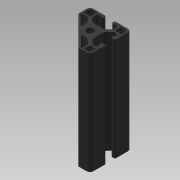
# Autodesk Inventor part: 40-4045-LITE-BLACK-FB
Saved by Autodesk Inventor 2013 (Build 170138000, 138)
## iProperties
Company: 80/20 Inc.
Created: 2014-04-23
Part Number: 40-4045-LITE-BLACK-FB
Material: Generic
Document SubType Name: Modeling
Designer: Ross Bowman
Density: 1 g/cm^3
Engineer: Ross Bowman
Catalog Web Link: 8020.net
Vendor: 80/20 Inc.
Material: 6105-T5 Aluminum
Author: Ross Bowman
Keywords: 80/20 , 8020 , T-Slot , Extrusion
Autodesk Inventor part; units mm, degrees
ref_plane "YZ Plane" through (0, 0, 0) normal (1, 0, 0) x (0, 1, 0)
ref_plane "XZ Plane" through (0, 0, 0) normal (0, 1, 0) x (-1, 0, 0)
ref_plane "XY Plane" through (0, 0, 0) normal (0, 0, 1) x (1, 0, 0)
sketch "Sketch1" plane through (0, 0, 0) normal (0, 0, 1) x (1, 0, 0)
  circle A0 centre (0, 0) radius 3.4
  arc A1 (-13.205, 12.2693) -> (-11.935, 13.5393) centre (-13.205, 13.5393) ccw
  line L0 (-17.695, 12.2693) -> (-13.205, 12.2693)
  arc A2 (-18.325, 12.8993) -> (-17.695, 12.2693) centre (-17.695, 12.8993) ccw
  line L1 (-18.325, 15.8793) -> (-18.325, 12.8993)
  arc A3 (-15.525, 18.6793) -> (-18.325, 15.8793) centre (-15.525, 15.8793) ccw
  line L2 (-12.565, 18.6793) -> (-15.525, 18.6793)
  arc A4 (-11.935, 18.0493) -> (-12.565, 18.6793) centre (-12.565, 18.0493) ccw
  line L3 (-11.935, 13.5393) -> (-11.935, 18.0493)
  arc A5 (-7.7004, 3.4003) -> (-9.0909, 6.7575) centre (-12.4481, 3.4003) ccw
  line L4 (-7.7004, 0.5997) -> (-7.7004, 3.4003)
  arc A6 (-8.9978, 0.0623) -> (-7.7004, 0.5997) centre (-8.4604, 0.5997) ccw
  line L5 (-18.2574, 9.3219) -> (-8.9978, 0.0623)
  arc A7 (-17.72, 10.6193) -> (-18.2574, 9.3219) centre (-17.72, 9.8593) ccw
  line L6 (-13.3072, 10.6193) -> (-17.72, 10.6193)
  arc A8 (-12.7021, 10.3687) -> (-13.3072, 10.6193) centre (-13.3072, 9.7636) ccw
  line L7 (-9.0909, 6.7575) -> (-12.7021, 10.3687)
  arc A9 (10.5703, -13.2185) -> (10.3477, -12.6811) centre (9.8103, -13.2185) ccw
  line L8 (10.5703, -17.6313) -> (10.5703, -13.2185)
  arc A10 (9.2729, -18.1687) -> (10.5703, -17.6313) centre (9.8103, -17.6313) ccw
  line L9 (-0.0445, -8.8513) -> (9.2729, -18.1687)
  arc A11 (0.4929, -7.5539) -> (-0.0445, -8.8513) centre (0.4929, -8.3139) ccw
  line L10 (3.2583, -7.5539) -> (0.4929, -7.5539)
  arc A12 (6.6079, -8.9413) -> (3.2583, -7.5539) centre (3.2583, -12.2908) ccw
  line L11 (10.3477, -12.6811) -> (6.6079, -8.9413)
  arc A13 (12.2693, -17.72) -> (12.8993, -18.35) centre (12.8993, -17.72) ccw
  line L12 (12.2693, -13.5393) -> (12.2693, -17.72)
  arc A14 (13.5393, -12.2693) -> (12.2693, -13.5393) centre (13.5393, -13.5393) ccw
  line L13 (17.72, -12.2693) -> (13.5393, -12.2693)
  arc A15 (18.35, -12.8993) -> (17.72, -12.2693) centre (17.72, -12.8993) ccw
  line L14 (18.35, -15.55) -> (18.35, -12.8993)
  arc A16 (15.55, -18.35) -> (18.35, -15.55) centre (15.55, -15.55) ccw
  line L15 (12.8993, -18.35) -> (15.55, -18.35)
  arc A17 (12.565, 18.332) -> (11.935, 17.702) centre (12.565, 17.702) ccw
  line L16 (15.55, 18.332) -> (12.565, 18.332)
  arc A18 (18.35, 15.532) -> (15.55, 18.332) centre (15.55, 15.532) ccw
  line L17 (18.35, 12.8413) -> (18.35, 15.532)
  arc A19 (17.745, 12.2693) -> (18.35, 12.8413) centre (17.7226, 12.8989) ccw
  line L18 (13.205, 12.2693) -> (17.745, 12.2693)
  arc A20 (11.935, 13.5393) -> (13.205, 12.2693) centre (13.205, 13.5393) ccw
  line L19 (11.935, 17.702) -> (11.935, 13.5393)
  arc A21 (8.04, -3.74) -> (9.4306, -7.0971) centre (12.7878, -3.74) ccw
  line L20 (8.04, -3.74) -> (8.04, 3.74)
  arc A22 (9.4306, 7.0971) -> (8.04, 3.74) centre (12.7878, 3.74) ccw
  line L21 (9.4306, 7.0971) -> (12.6921, 10.3586)
  arc A23 (13.3214, 10.6193) -> (12.6921, 10.3586) centre (13.3214, 9.7293) ccw
  line L22 (13.3214, 10.6193) -> (14.8088, 10.6193)
  arc A24 (16.7, 8.7281) -> (14.8088, 10.6193) centre (14.8088, 8.7281) ccw
  line L23 (16.7, 8.7281) -> (16.7, 6.9134)
  line L24 (16.7, 6.9134) -> (15.94, 6.9134)
  line L25 (15.94, 6.9134) -> (15.94, 5.7595)
  arc A25 (15.94, 5.7595) -> (17.51, 4.1895) centre (17.51, 5.7595) ccw
  line L26 (17.51, 4.1895) -> (18.43, 4.1895)
  arc A26 (18.43, 4.1895) -> (20, 5.7595) centre (18.43, 5.7595) ccw
  line L27 (20, 5.7595) -> (20, 16.8689)
  arc A27 (20, 16.8689) -> (16.8881, 20) centre (16.8302, 16.8305) ccw
  line L28 (16.8881, 20) -> (5.6295, 20)
  arc A28 (5.6295, 20) -> (4.06, 18.4701) centre (5.6295, 18.43) ccw
  line L29 (4.06, 18.4701) -> (4.06, 17.5501)
  arc A29 (4.06, 17.5501) -> (5.63, 16.8567) centre (5.3762, 18.406) ccw
  line L30 (5.63, 16.8567) -> (6.7535, 16.8567)
  line L31 (6.7535, 16.8567) -> (6.7535, 17.6167)
  line L32 (6.7535, 17.6167) -> (8.3698, 17.6167)
  arc A30 (10.285, 15.7015) -> (8.3698, 17.6167) centre (8.3698, 15.7015) ccw
  line L33 (10.285, 15.7015) -> (10.285, 12.8154)
  arc A31 (10.2371, 12.5705) -> (10.285, 12.8154) centre (9.6352, 12.8154) ccw
  line L34 (10.2371, 12.5705) -> (7.0971, 9.4306)
  arc A32 (3.74, 8.04) -> (7.0971, 9.4306) centre (3.74, 12.7878) ccw
  line L35 (3.74, 8.04) -> (-3.74, 8.04)
  arc A33 (-7.0971, 9.4306) -> (-3.74, 8.04) centre (-3.74, 12.7878) ccw
  line L36 (-7.0971, 9.4306) -> (-10.0289, 12.3623)
  arc A34 (-10.285, 12.9807) -> (-10.0289, 12.3623) centre (-9.4106, 12.9807) ccw
  line L37 (-10.285, 12.9807) -> (-10.285, 15.7015)
  arc A35 (-8.3698, 17.6167) -> (-10.285, 15.7015) centre (-8.3698, 15.7015) ccw
  line L38 (-8.3698, 17.6167) -> (-6.7535, 17.6167)
  line L39 (-6.7535, 17.6167) -> (-6.7535, 16.8567)
  line L40 (-6.7535, 16.8567) -> (-5.63, 16.8567)
  arc A36 (-5.63, 16.8567) -> (-4.06, 18.4267) centre (-5.63, 18.4267) ccw
  line L41 (-4.06, 18.4267) -> (-4.06, 18.4153)
  arc A37 (-4.06, 18.4153) -> (-5.6299, 20) centre (-5.6299, 18.43) ccw
  line L42 (-5.6299, 20) -> (-16.83, 20)
  arc A38 (-16.83, 20) -> (-20, 16.83) centre (-16.83, 16.83) ccw
  line L43 (-20, 16.83) -> (-20, 9.3524)
  arc A39 (-20, 9.3524) -> (-19.5607, 8.2917) centre (-18.5, 9.3524) ccw
  line L44 (-19.5607, 8.2917) -> (8.2917, -19.5607)
  arc A40 (8.2917, -19.5607) -> (9.3524, -20) centre (9.3524, -18.5) ccw
  line L45 (9.3524, -20) -> (16.83, -20)
  arc A41 (16.83, -20) -> (20, -16.83) centre (16.83, -16.83) ccw
  line L46 (20, -16.83) -> (20, -5.7595)
  arc A42 (20, -5.7595) -> (18.43, -4.1895) centre (18.43, -5.7595) ccw
  line L47 (18.43, -4.1895) -> (17.51, -4.1895)
  arc A43 (17.51, -4.1895) -> (15.94, -5.7595) centre (17.51, -5.7595) ccw
  line L48 (15.94, -5.7595) -> (15.94, -6.9134)
  line L49 (15.94, -6.9134) -> (16.7, -6.9134)
  line L50 (16.7, -6.9134) -> (16.7, -8.7281)
  arc A44 (14.8088, -10.6193) -> (16.7, -8.7281) centre (14.8088, -8.7281) ccw
  line L51 (14.8088, -10.6193) -> (13.3214, -10.6193)
  arc A45 (12.6921, -10.3586) -> (13.3214, -10.6193) centre (13.3214, -9.7293) ccw
  line L52 (12.6921, -10.3586) -> (9.4306, -7.0971)
  constraints: 106 end point, 90 point on circle, 46 centre point
extrude "Extrusion1" add sketch "Sketch1" against normal blind 100
body "Solid1"
